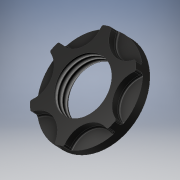
# Autodesk Inventor part: Part2
Saved by Autodesk Inventor 2019 (Build 230136000, 136)
## iProperties
Created: 2021-05-14
Part Number: Part2
Material: Generic
Document SubType Name: Modeling
Designer: HP
Density: 1 g/cm^3
Appearance: Default
Author: HP
Autodesk Inventor part; units mm, degrees
ref_plane "YZ Plane" through (0, 0, 0) normal (1, 0, 0) x (0, 1, 0)
ref_plane "XZ Plane" through (0, 0, 0) normal (0, 1, 0) x (-1, 0, 0)
ref_plane "XY Plane" through (0, 0, 0) normal (0, 0, 1) x (1, 0, 0)
sketch "Sketch1" plane through (0, 0, 0) normal (0, 0, 1) x (1, 0, 0)
  circle A0 centre (0, 0) radius 27.5
  circle A1 centre (0, 0) radius 15
  dimension "d0" = 55
  dimension "d1" = 30
  constraints: 2 centre point, 2 coincident
  measures "d0" diameter of A0
  measures "d1" diameter of A1
extrude "Extrusion1" add sketch "Sketch1" along normal blind 10
sketch "Sketch2" plane through (0, 0, 10) normal (0, 0, 1) x (1, 0, 0)
  circle A0 centre (0, 0) radius 27.5
  arc A1 (-10.874, 25.258783) -> (11.632095, 24.918755) centre (0.473516, 31.341506) ccw
  constraints: 4 point on circle, 1 centre point
extrude "Extrusion2" cut sketch "Sketch2" against normal blind 5 contours A1 A0 picked at (3.778626, 24.499715)
fillet "Fillet1" radius 1 3 edges at (0.279, 18.468, 5) (-10.874, 25.2588, 7.5) (11.6321, 24.9188, 7.5)
pattern_circular "Circular Pattern1" count 6 over 360 about axis through (0, 0, 0) along (0, 0, 1) of "Extrusion2", "Fillet1"
thread "Thread1" size "M30x3.5" class "6H" standard "ANSI Metric M Profile" full length
body "Solid1"
